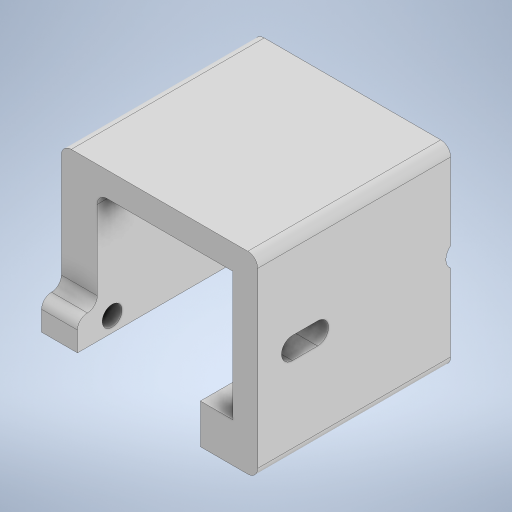
# Autodesk Inventor part: camera_lock
Saved by Autodesk Inventor 2024 (Build 280153000, 153)
## iProperties
Created: 2024-07-18
Part Number: camera_lock
Material: Generic
Document SubType Name: Modeling
Designer: mamof
Density: 1 g/cm^3
Appearance: Default
Author: mamof
Autodesk Inventor part; units mm, degrees
ref_plane "YZ Plane" through (0, 0, 0) normal (1, 0, 0) x (0, 1, 0)
ref_plane "XZ Plane" through (0, 0, 0) normal (0, 1, 0) x (-1, 0, 0)
ref_plane "XY Plane" through (0, 0, 0) normal (0, 0, 1) x (1, 0, 0)
sketch "Sketch1" plane through (0, 0, 0) normal (1, 0, 0) x (0, 1, 0)
  line L0 (0, 0) -> (0, 23.5)
  line L1 (0, 23.5) -> (6, 23.5)
  line L2 (6, 23.5) -> (6, -23.5)
  line L3 (6, -23.5) -> (0, -23.5)
  line L4 (0, -23.5) -> (0, 0)
  line L5 (6, 23.5) -> (6, 21.5)
  line L6 (6, 21.5) -> (4, 21.5)
  circle A0 centre (4, 21.5) radius 2
  line L7 (6, -23.5) -> (6, -21.5)
  line L8 (6, -21.5) -> (4, -21.5)
  circle A1 centre (4, -21.5) radius 2
  line L9 (6, -23.5) -> (6, -16.5)
  line L10 (6, -16.5) -> (3, -16.5)
  line L11 (6, 23.5) -> (6, 16.5)
  line L12 (6, 16.5) -> (3, 16.5)
  circle A2 centre (3, 16.5) radius 2
  circle A3 centre (3, -16.5) radius 2
  point P0 (4, 23.5)
  point P1 (4, -23.5)
  dimension "d0" = 23.5
  dimension "d1" = 6
  dimension "d2" = 47
  dimension "d3" = 6
  dimension "d4" = 2
  dimension "d5" = 2
  dimension "d6" = 4
  dimension "d7" = 2
  dimension "d8" = 2
  dimension "d9" = 4
  dimension "d10" = 7
  dimension "d11" = 3
  dimension "d12" = 7
  dimension "d13" = 3
  dimension "d14" = 4
  dimension "d15" = 4
  constraints: 26 end point, 6 perpendicular, 5 point on line, 4 centre point, 4 coincident, 1 collinear, 1 vertical
  measures "d0" distance of L0.start L0.end
  measures "d1" distance of L0.end L1.end
  measures "d2" distance of L1.end L2.end
  measures "d3" distance of L2.end L3.end
  measures "d4" distance of L1.end L5.end
  measures "d5" distance of L5.end L6.end
  measures "d6" diameter of A0
  measures "d7" distance of L2.end L7.end
  measures "d8" distance of L7.end L8.end
  measures "d9" diameter of A1
  measures "d10" distance of L2.end L9.end
  measures "d11" distance of L9.end L10.end
  measures "d12" distance of L1.end L11.end
  measures "d13" distance of L11.end L12.end
  measures "d14" diameter of A2
  measures "d15" diameter of A3
extrude "Extrusion1" add sketch "Sketch1" along normal blind 7.2555 contours L0 L1 A0 L2 A1 L3 L4 | A0 | A1
sketch "Sketch2" plane through (0, 6, 21.5) normal (0, 1, 0) x (1, 0, 0)
  line L0 (7.2555, -2) -> (7.2555, 0) projected
  line L1 (0, 0) -> (7.2555, 0) projected
  line L2 (7.2555, 0) -> (0, 0)
  line L3 (0, 0) -> (0, 43)
  line L4 (0, -2) -> (0, 45) projected
  line L5 (0, 43) -> (7.2555, 43)
  line L6 (7.2555, 43) -> (7.2555, 0)
  point P0 (0, 21.5)
  dimension "d18" = 7.2555
  dimension "d19" = 43
  dimension "d20" = 7.2555
  constraints: 8 end point, 1 horizontal, 1 perpendicular, 1 point on line
  measures "d18" distance of L0.end L1.start
  measures "d19" distance of L1.start L3.end
  measures "d20" distance of L3.end L5.end
extrude "Extrusion2" add sketch "Sketch2" along normal blind 25
sketch "Sketch3" plane through (0, 0, 0) normal (-1, 0, 0) x (0, 0, 1)
  arc A0 (23.5, 4) -> (21.5, 6) centre (21.5, 4) ccw projected
  line L0 (21.5, 6) -> (21.5, 8)
  line L1 (21.5, 6) -> (21.5, 31) projected
  circle A1 centre (21.5, 8) radius 2
  line L2 (19.5, 8) -> (19.5, 31)
  line L3 (21.5, 31) -> (-21.5, 31) projected
  line L4 (19.5, 31) -> (21.5, 31)
  line L5 (21.5, 31) -> (21.5, 10)
  line L6 (-21.5, 6) -> (-21.5, 31) projected
  line L7 (-21.5, 6) -> (-21.5, 8)
  circle A2 centre (-21.5, 8) radius 2
  line L8 (-19.5, 8) -> (-19.5, 31)
  line L9 (-19.5, 31) -> (-21.5, 31)
  line L10 (-21.5, 31) -> (-21.5, 10)
  point P0 (0, 0)
  dimension "d23" = 2
  dimension "d24" = 4
  dimension "d25" = 23
  dimension "d26" = 2
  dimension "d27" = 4
  dimension "d28" = 23
  constraints: 16 end point, 6 point on line, 4 point on circle, 2 centre point, 2 coincident, 1 collinear, 1 perpendicular
  measures "d23" distance of L0.start L0.end
  measures "d24" diameter of A1
  measures "d25" distance of L2.start L2.end
  measures "d26" distance of L6.start L7.end
  measures "d27" diameter of A2
  measures "d28" distance of L8.start L8.end
extrude "Extrusion3" cut sketch "Sketch3" against normal blind 7.2555 contours A1 L1 L0 | L8 A2 L6 L3 | L2 L3 L1 A1 | A2 L6 picked at (20.5631, 8.9369) picked at (-20.5631, 7.0631)
sketch "Sketch4" plane through (7.2555, 0, 0) normal (1, 0, 0) x (0, 0, -1)
  line L0 (-19.5, 31) -> (19.5, 31) projected
  line L1 (-19.5, 31) -> (-19.5, 26)
  line L2 (-19.5, 8) -> (-19.5, 31) projected
  line L3 (-19.5, 26) -> (19.5, 26)
  line L4 (19.5, 26) -> (19.5, 31)
  line L5 (-19.5, 31) -> (19.5, 31)
  point P0 (0, 0)
  dimension "d31" = 5
  dimension "d32" = 39
  constraints: 8 end point, 1 collinear, 1 horizontal, 1 point on line
  measures "d31" distance of L0.start L1.end
  measures "d32" distance of L1.end L3.end
extrude "Extrusion4" add sketch "Sketch4" along normal blind 27.422
sketch "Sketch5" plane through (0, 8, 19.5) normal (0, 0, 1) x (1, 0, 0)
  line L0 (0, 0) -> (0, 23) projected
  line L1 (0, 23) -> (0, 21)
  line L2 (0, 21) -> (2, 21)
  circle A0 centre (2, 21) radius 2
  line L3 (0, 23) -> (2, 23)
  line L4 (0, 23) -> (34.6775, 23) projected
  line L5 (7.2555, 18) -> (34.6775, 18) projected
  line L6 (7.2555, 18) -> (7.2555, 16)
  line L7 (7.2555, 16) -> (9.2555, 16)
  circle A1 centre (9.2555, 16) radius 2
  line L8 (7.2555, 18) -> (9.2555, 18)
  point P0 (0, -8)
  point P1 (7.2555, 16)
  dimension "d37" = 4
  dimension "d40" = 4
  dimension "d35" = 2
  dimension "d36" = 2
  dimension "d38" = 2
  dimension "d39" = 2
  constraints: 12 end point, 3 point on line, 2 coincident, 2 perpendicular, 1 vertical, 6 other
  measures "d35" distance of L0.end L1.end
  measures "d36" distance of L1.end L2.end
  measures "d38" distance of L5.start L6.end
  measures "d39" distance of L6.end L7.end
extrude "Extrusion5" cut sketch "Sketch5" against normal blind 39 contours L0 L3 A0 | L5 A1 L6
sketch "Sketch6" plane through (0, 8, 19.5) normal (0, 0, 1) x (1, 0, 0)
  line L0 (7.2555, 18) -> (7.2555, 0) projected
  line L1 (7.2555, 18) -> (7.2555, 16)
  line L2 (7.2555, 16) -> (9.2555, 16)
  circle A0 centre (9.2555, 16) radius 2
  line L3 (7.2555, 18) -> (34.6775, 18) projected
  line L4 (7.2555, 18) -> (9.2555, 18)
  point P0 (0, -8)
  point P1 (7.2555, 16)
  dimension "d45" = 4
  dimension "d43" = 2
  dimension "d44" = 2
  constraints: 6 end point, 2 point on line, 1 coincident, 1 perpendicular, 3 other
  measures "d43" distance of L0.start L1.end
  measures "d44" distance of L1.end L2.end
extrude "Extrusion6" add sketch "Sketch6" against normal blind 39 contours L3 A0 L0
sketch "Sketch7" plane through (34.6775, 0, 0) normal (1, 0, 0) x (0, 0, -1)
  line L0 (-19.5, 31) -> (-19.5, 26) projected
  line L1 (19.5, 26) -> (19.5, 31) projected
  line L2 (-19.5, 31) -> (19.5, 31)
  line L3 (19.5, 31) -> (19.5, 26)
  line L4 (19.5, 26) -> (-19.5, 26)
  line L5 (-19.5, 26) -> (-19.5, 31)
  point P0 (0, 0)
  constraints: 8 end point, 2 perpendicular, 1 collinear, 1 horizontal
extrude "Extrusion7" add sketch "Sketch7" along normal blind 5
sketch "Sketch8" plane through (0, 8, 19.5) normal (0, 0, 1) x (1, 0, 0)
  line L0 (39.6775, 23) -> (2, 23) projected
  line L1 (39.6775, 23) -> (37.6775, 23)
  line L2 (37.6775, 23) -> (37.6775, 21)
  circle A0 centre (37.6775, 21) radius 2
  line L3 (39.6775, 23) -> (39.6775, 21)
  point P0 (0, -8)
  dimension "d52" = 4
  dimension "d50" = 2
  dimension "d51" = 2
  constraints: 6 end point, 1 coincident, 1 perpendicular, 1 point on line, 1 vertical, 3 other
  measures "d50" distance of L0.start L1.end
  measures "d51" distance of L1.end L2.end
extrude "Extrusion8" cut sketch "Sketch8" against normal blind 39 contours L3 A0 L0
sketch "Sketch9" plane through (9.2555, 26, -19.5) normal (0, -1, 0) x (1, 0, 0)
  line L0 (30.422, 39) -> (30.422, 0) projected
  line L1 (30.422, 39) -> (25.422, 39)
  line L2 (0, 39) -> (30.422, 39) projected
  line L3 (25.422, 39) -> (25.422, 0)
  line L4 (25.422, 0) -> (30.422, 0)
  line L5 (30.422, 0) -> (30.422, 39)
  point P0 (-9.2555, 19.5)
  dimension "d55" = 5
  dimension "d56" = 39
  constraints: 8 end point, 3 perpendicular, 1 point on line
  measures "d55" distance of L0.start L1.end
  measures "d56" distance of L1.end L3.end
extrude "Extrusion9" add sketch "Sketch9" along normal blind 34
sketch "Sketch10" plane through (39.6775, 0, 0) normal (1, 0, 0) x (0, 0, -1)
  line L0 (-19.5, 31) -> (-19.5, 29) projected
  line L1 (-19.5, 29) -> (-19.5, 26)
  line L2 (-19.5, 29) -> (-19.5, -8) projected
  line L3 (-19.5, 26) -> (19.5, 26)
  line L4 (19.5, 26) -> (19.5, 29)
  line L5 (19.5, 29) -> (-19.5, 29)
  line L6 (-19.5, 26) -> (-9.933, 26)
  line L7 (-9.933, 26) -> (-9.933, 13.756)
  line L8 (-9.933, 13.756) -> (-7.383, 13.756)
  line L9 (-7.383, 13.756) -> (-7.383, 11.556)
  line L10 (-7.383, 11.556) -> (-7.383, 9.356)
  line L11 (-7.383, 9.356) -> (-12.483, 9.356)
  line L12 (-12.483, 9.356) -> (-12.483, 11.556)
  line L13 (-12.483, 11.556) -> (-12.483, 13.756)
  line L14 (-12.483, 13.756) -> (-9.933, 13.756)
  circle A0 centre (-7.383, 11.556) radius 2.2
  circle A1 centre (-12.483, 11.556) radius 2.2
  line L15 (19.5, 26) -> (21.044, 26)
  line L16 (21.044, 26) -> (21.044, 11.5)
  circle A2 centre (21.044, 11.5) radius 2.5
  point P0 (0, 0)
  dimension "d59" = 3
  dimension "d60" = 39
  dimension "d61" = 9.567
  dimension "d62" = 12.244
  dimension "d63" = 2.55
  dimension "d64" = 2.2
  dimension "d65" = 2.2
  dimension "d66" = 5.1
  dimension "d67" = 2.2
  dimension "d68" = 2.2
  dimension "d69" = 4.4
  dimension "d70" = 4.4
  dimension "d71" = 1.544
  dimension "d72" = 14.5
  dimension "d73" = 5
  constraints: 30 end point, 7 perpendicular, 4 point on line, 3 centre point, 3 coincident, 1 horizontal, 1 parallel, 1 vertical
  measures "d59" distance of L0.end L1.end
  measures "d60" distance of L1.end L3.end
  measures "d61" distance of L1.end L6.end
  measures "d62" distance of L6.end L7.end
  measures "d63" distance of L7.end L8.end
  measures "d64" distance of L8.end L9.end
  measures "d65" distance of L9.end L10.end
  measures "d66" distance of L10.end L11.end
  measures "d67" distance of L11.end L12.end
  measures "d68" distance of L12.end L13.end
  measures "d69" diameter of A0
  measures "d70" diameter of A1
  measures "d71" distance of L3.end L15.end
  measures "d72" distance of L15.end L16.end
  measures "d73" diameter of A2
extrude "Extrusion10" cut sketch "Sketch10" against normal blind 5 contours A2 | L8 A0 L11 A1 L14 | A0 L10 L9 | L9 L10 A0 | A1 L12 L13 | L13 L12 A1
sketch "Sketch11" plane through (34.6775, 26, -19.5) normal (-1, 0, 0) x (0, 0, 1)
  line L0 (39, -34) -> (0, -34) projected
  line L1 (39, -34) -> (39, -26)
  line L2 (39, 3) -> (39, -34) projected
  line L3 (39, -26) -> (0, -26)
  line L4 (0, -26) -> (0, -34)
  line L5 (0, -34) -> (39, -34)
  point P0 (19.5, -26)
  dimension "d76" = 8
  dimension "d77" = 39
  constraints: 8 end point, 3 perpendicular, 1 point on line
  measures "d76" distance of L0.start L1.end
  measures "d77" distance of L1.end L3.end
extrude "Extrusion11" add sketch "Sketch11" along normal blind 6.58
sketch "Sketch12" plane through (0, 8, 19.5) normal (0, 0, 1) x (1, 0, 0)
  line L0 (39.6775, 21) -> (39.6775, -16) projected
  line L1 (39.6775, -16) -> (37.6775, -16)
  line L2 (39.6775, -16) -> (28.0975, -16) projected
  line L3 (37.6775, -16) -> (37.6775, -14)
  circle A0 centre (37.6775, -14) radius 2
  line L4 (39.6775, -16) -> (39.6775, -14)
  point P0 (0, -8)
  point P1 (37.6775, -16)
  dimension "d82" = 4
  dimension "d80" = 2
  dimension "d81" = 2
  constraints: 6 end point, 2 point on line, 1 coincident, 1 perpendicular, 3 other
  measures "d80" distance of L0.end L1.end
  measures "d81" distance of L1.end L3.end
extrude "Extrusion12" cut sketch "Sketch12" against normal blind 39 contours L0 L1 A0
body "Solid1"
